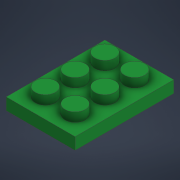
# Autodesk Inventor part: 110033226_ipt_02_草地一
Saved by Autodesk Inventor 2022 (Build 260153000, 153)
## iProperties
Created: 2022-06-22
Part Number: 110033226_ipt_02_草地一
Material: 一般
Document SubType Name: Modeling
Designer: User
Density: 1 g/cm^3
Appearance: 預設
Author: User
Autodesk Inventor part; units mm, degrees
ref_plane "YZ Plane" through (0, 0, 0) normal (1, 0, 0) x (0, 1, 0)
ref_plane "XZ Plane" through (0, 0, 0) normal (0, 1, 0) x (-1, 0, 0)
ref_plane "XY Plane" through (0, 0, 0) normal (0, 0, 1) x (1, 0, 0)
sketch "草圖1" plane through (0, 0, 0) normal (0, 1, 0) x (-1, 0, 0)
  line L0 (5.8, 8.3) -> (-5.8, 8.3)
  line L1 (-5.8, 8.3) -> (-5.8, -8.3)
  line L2 (-5.8, -8.3) -> (5.8, -8.3)
  line L3 (5.8, -8.3) -> (5.8, 8.3)
  point P0 (0, 0)
  point P1 (5.8, 0)
  point P2 (0, -8.3)
  dimension "d0" = 11.6
  dimension "d1" = 16.6
  constraints: 8 end point, 2 midpoint, 2 parallel, 1 horizontal, 1 horizontal alignment, 1 perpendicular, 1 vertical alignment
  measures "d0" distance of L2.end L1.end
  measures "d1" distance of L1.end L0.end
extrude "擠出1" add sketch "草圖1" along normal blind 2
sketch "草圖2" plane through (0, 0, 0) normal (0, -1, 0) x (1, 0, 0)
  line L0 (5.8, 8.3) -> (5.8, -8.3) projected
  line L1 (-5.8, 8.3) -> (5.8, 8.3) projected
  line L2 (-5.8, -8.3) -> (-5.8, 8.3) projected
  line L3 (5.8, -8.3) -> (-5.8, -8.3) projected
  circle A0 centre (2.5, 5) radius 1.7
  circle A1 centre (2.5, 5) radius 2.5
  point P0 (0, 0)
  dimension "d4" = 3.4
  dimension "d5" = 5
  dimension "d6" = 3.3
  dimension "d7" = 3.3
  constraints: 2 centre point, 1 coincident
  measures "d4" diameter of A0
  measures "d5" diameter of A1
  measures "d6" distance from line of L0 A0.centre
  measures "d7" distance from line of L1 A0.centre
extrude "擠出2" cut sketch "草圖2" against normal blind 1.5 contours A0
pattern_linear "矩形陣列1" count 3 spacing 5 along (0, 0, -1) count 2 spacing 5 along (-1, 0, 0) of "擠出2"
sketch "草圖3" plane through (0, 2, 0) normal (0, 1, 0) x (1, 0, 0)
  circle A0 centre (2.5, -5) radius 1.7
  line L0 (5.8, -8.3) -> (5.8, 8.3) projected
  line L1 (-5.8, -8.3) -> (5.8, -8.3) projected
  point P0 (0, 0)
  dimension "d16" = 3.4
  dimension "d17" = 3.3
  dimension "d18" = 3.3
  constraints: 1 centre point
  measures "d16" diameter of A0
  measures "d17" distance from line of L0 A0.centre
  measures "d18" distance from line of L1 A0.centre
extrude "擠出3" add sketch "草圖3" along normal blind 1.5
pattern_linear "矩形陣列2" count 3 spacing 5 along (0, 0, -1) count 2 spacing 5 along (-1, 0, 0) of "擠出3"
